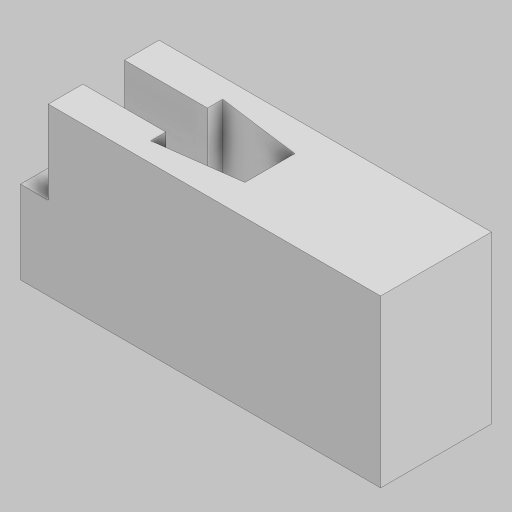
# Autodesk Inventor part: Tenon_Hembra_Parametrizada
Saved by Autodesk Inventor 2023 (Build 270158000, 158)
## iProperties
Created: 2026-02-15
Part Number: Tenon_Hembra_Parametrizada
Material: Genérico
Document SubType Name: Modeling
Designer: MARTIN MAESTRE
Density: 1 g/cm^3
Appearance: Valor por defecto
Author: MARTIN MAESTRE
Autodesk Inventor part; units mm, degrees
ref_plane "YZ Plane" through (0, 0, 0) normal (1, 0, 0) x (0, 1, 0)
ref_plane "XZ Plane" through (0, 0, 0) normal (0, 1, 0) x (-1, 0, 0)
ref_plane "XY Plane" through (0, 0, 0) normal (0, 0, 1) x (1, 0, 0)
sketch "Boceto1" plane through (0, 0, 0) normal (0, 0, 1) x (1, 0, 0)
  line L0 (0, 0) -> (70, 0)
  line L1 (70, 0) -> (130, 0)
  line L2 (0, 0) -> (0, 60)
  line L3 (0, 60) -> (130, 60)
  line L4 (130, 60) -> (130, 0)
  dimension "d0" = 70
  dimension "d1" = 60
  dimension "d2" = 60
  constraints: 10 end point, 2 horizontal, 2 perpendicular, 1 vertical
  measures "d0" distance of L0.start L0.end
  measures "d1" distance of L0.end L1.end
  measures "d2" distance of L0.start L2.end
extrude "Extrusión1" add sketch "Boceto1" along normal blind 40
sketch "Boceto2" plane through (0, 60, 0) normal (0, 1, 0) x (1, 0, 0)
  line L0 (0, 0) -> (130, 0) projected
  line L1 (0, 0) -> (0, -40)
  line L2 (0, 0) -> (10, 0)
  line L3 (0, 0) -> (10, 0) construction
  line L4 (10, 0) -> (10, -40)
  line L5 (10, -40) -> (0, -40)
  line L6 (10, 0) -> (10, -12.5) construction
  line L7 (10, -12.5) -> (40, -12.5)
  line L8 (40, -12.5) -> (40, -7)
  line L9 (10, -12.5) -> (10, -27.5) construction
  line L10 (10, -27.5) -> (40, -27.5)
  line L11 (40, -27.5) -> (40, -33)
  line L12 (10, -12.5) -> (70, -12.5) construction
  line L13 (70, -12.5) -> (70, -11)
  line L14 (70, -12.5) -> (70, -29)
  line L15 (70, -29) -> (40, -33)
  line L16 (40, -7) -> (70, -11)
  dimension "d5" = 10
  dimension "d6" = 0
  dimension "d7" = 40
  dimension "d8" = 12.5
  dimension "d9" = 30
  dimension "d10" = 5.5
  dimension "d11" = 15
  dimension "d12" = 5.5
  dimension "d13" = 30
  dimension "d14" = 60
  dimension "d15" = 1.5
  dimension "d16" = 16.5
  constraints: 32 end point, 5 vertical, 3 horizontal, 3 point on line, 2 collinear, 2 perpendicular
  measures "d5" distance of L0.start L2.end
  measures "d6" distance between parallel lines of L2 L3
  measures "d7" distance between parallel lines of L3 L5
  measures "d8" distance of L3.end L6.end
  measures "d9" distance of L6.end L7.end
  measures "d10" distance of L7.end L8.end
  measures "d11" distance of L6.end L9.end
  measures "d12" distance of L10.end L11.end
  measures "d13" distance between parallel lines of L4 L11
  measures "d14" distance of L6.end L12.end
  measures "d15" distance of L12.end L13.end
  measures "d16" distance of L12.end L14.end
extrude "Extrusión2" cut sketch "Boceto2" against normal blind 30
equation "\"d3\" = Profundidad"
equation "\"d5\" = Separación_lateral"
equation "\"d8\" = Separacion_superior"
equation "\"d10\" = Rebaje_superior"
equation "\"d12\" = Rebaje_inferior"
equation "\"d15\" = Espesor_detalle"
equation "\"d16\" = Distancia_centro"
equation "\"Profundidad\" = 40 * Escala"
equation "\"Rebaje_superior\" = 5.5 * Escala"
equation "\"Rebaje_inferior\" = 5.5 * Escala"
equation "\"Separacion_superior\" = 12.5 * Escala"
equation "\"Separación_lateral\" = Escala"
equation "\"Distancia_centro\" = 16.5 * Escala"
equation "\"Espesor_detalle\" = 1.5 * Escala"
equation "\"Escala\" = 1"
